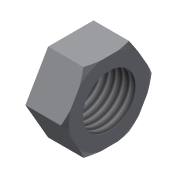
# Autodesk Inventor part: Nut3
Saved by Autodesk Inventor 2022.5 (Build 265521000, 521)
## iProperties
Created: 2011-08-19
Part Number: Nut3
Document SubType Name: Modeling
Designer: nguyenducthang
Density: 1 g/cm^3
Mass: 0.0230266 g
Surface Area: 0.754722 cm^2
Volume: 0.0230266 cm^3
Material: Generic
Appearance: Default
Author: nguyenducthang
Autodesk Inventor part; units mm, degrees
ref_plane "YZ Plane" through (0, 0, 0) normal (1, 0, 0) x (0, 1, 0)
ref_plane "XZ Plane" through (0, 0, 0) normal (0, 1, 0) x (-1, 0, 0)
ref_plane "XY Plane" through (0, 0, 0) normal (0, 0, 1) x (1, 0, 0)
sketch "Sketch17" plane through (0, 0, 0) normal (0, 0, 1) x (1, 0, 0)
  line L0 (0, 0) -> (0, 2.6) construction
  line L1 (0, 2.6) -> (2.2, 2.6)
  line L2 (2.2, 2.6) -> (2.2, 1.5)
  line L3 (2.2, 1.5) -> (0, 1.5)
  line L4 (0, 0) -> (5.189, 0) construction
  line L5 (0, 1.5) -> (0, 2.6)
  dimension "d96" = 1.5
  dimension "d98" = 2.6
  dimension "d99" = 0
  dimension "d100" = 2.2
  constraints: 12 end point, 2 parallel, 1 collinear, 1 horizontal, 1 perpendicular, 1 point on line, 1 vertical, 1 other
  measures "d96" distance between parallel lines of L3 L4
  measures "d98" distance between parallel lines of L1 L4
  measures "d99" distance from line of L0 L4.start
  measures "d100" distance between parallel lines of L0 L2
revolve "Revolution3" add sketch "Sketch17" angle 360 about axis through (0, 0, 0) along (1, 0, 0)
chamfer "Chamfer2" distance 0.3 angle 30 1 edges at (2.2, -2.6, 0) measured on face at (2.2, 2.2081, -0.2074)
sketch "Sketch18" plane through (2.2, 0, 0) normal (1, 0, 0) x (0, 0, -1)
  circle A0 centre (0, 0) radius 2.3 construction
  line L0 (1.3, 2.2517) -> (2.6, 0)
  line L1 (2.6, 0) -> (1.3, -2.2517)
  line L2 (1.3, -2.2517) -> (-1.3, -2.2517)
  line L3 (-1.3, -2.2517) -> (-2.6, 0)
  line L4 (-2.6, 0) -> (-1.3, 2.2517)
  line L5 (-1.3, 2.2517) -> (1.3, 2.2517)
  circle A1 centre (0, 0) radius 5.5787
  dimension "d106" = 2.6
  constraints: 12 end point, 2 coincident, 1 centre point, 13 other
  measures "d106" distance of L1.end L2.end
extrude "Extrusion15" cut sketch "Sketch18" along normal through all both and the other way through all
thread "Thread2" size "M2x0.4" class "6H" standard "ANSI Metric M Profile" full length
body "Solid1"
